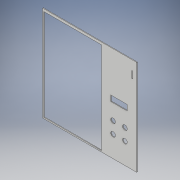
# Autodesk Inventor part: face-avant
Saved by Autodesk Inventor 2019 (Build 230136000, 136)
## iProperties
Created: 2018-12-30
Part Number: face-avant
Material: Générique
Document SubType Name: Modeling
Designer: pouey
Density: 1 g/cm^3
Appearance: Par défaut
Author: pouey
Autodesk Inventor part; units mm, degrees
ref_plane "YZ Plane" through (0, 0, 0) normal (1, 0, 0) x (0, 1, 0)
ref_plane "XZ Plane" through (0, 0, 0) normal (0, 1, 0) x (-1, 0, 0)
ref_plane "XY Plane" through (0, 0, 0) normal (0, 0, 1) x (1, 0, 0)
sketch "Esquisse1" plane through (0, 0, 0) normal (0, 0, 1) x (1, 0, 0)
  line L0 (0, 0) -> (400, 0)
  line L1 (400, 0) -> (400, 405)
  line L2 (400, 405) -> (0, 405)
  line L3 (0, 405) -> (0, 0)
  dimension "d0" = 400
  dimension "d1" = 405
  constraints: 8 end point, 2 parallel, 1 horizontal, 1 perpendicular
  measures "d0" distance of L1.end L2.end
  measures "d1" distance of L0.end L1.end
extrude "Extrusion1" add sketch "Esquisse1" along normal blind 3
sketch "Esquisse2" plane through (0, 0, 3) normal (0, 0, 1) x (1, 0, 0)
  line L0 (5, 395) -> (250, 395)
  line L1 (250, 395) -> (250, 5)
  line L2 (250, 5) -> (5, 5)
  line L3 (5, 5) -> (5, 395)
  line L4 (0, 0) -> (400, 0) projected
  line L5 (0, 405) -> (0, 0) projected
  dimension "d4" = 390
  dimension "d5" = 5
  dimension "d6" = 5
  dimension "d7" = 245
  constraints: 8 end point, 2 parallel, 1 horizontal, 1 perpendicular
  measures "d4" distance of L0.end L1.end
  measures "d5" distance between parallel lines of L4 L2
  measures "d6" distance between parallel lines of L5 L3
  measures "d7" distance between parallel lines of L3 L1
extrude "Extrusion2" cut sketch "Esquisse2" against normal blind 3
sketch "Esquisse3" plane through (0, 0, 3) normal (0, 0, 1) x (1, 0, 0)
  line L0 (290, 230) -> (360, 230)
  line L1 (360, 230) -> (360, 206)
  line L2 (360, 206) -> (290, 206)
  line L3 (290, 206) -> (290, 230)
  line L4 (250, 395) -> (250, 5) projected
  line L5 (400, 405) -> (0, 405) projected
  circle A0 centre (300, 140) radius 10
  circle A1 centre (350, 140) radius 10
  circle A2 centre (300, 90) radius 10
  circle A3 centre (350, 90) radius 10
  line L6 (0, 0) -> (400, 0) projected
  dimension "d10" = 24
  dimension "d11" = 70
  dimension "d13" = 40
  dimension "d14" = 175
  dimension "d17" = 20
  dimension "d18" = 20
  dimension "d19" = 20
  dimension "d20" = 20
  dimension "d21" = 50
  dimension "d22" = 100
  dimension "d23" = 140
  dimension "d24" = 140
  dimension "d25" = 50
  dimension "d26" = 90
  dimension "d27" = 90
  dimension "d28" = 100
  constraints: 8 end point, 4 centre point, 2 parallel, 1 horizontal, 1 perpendicular
  measures "d10" distance of L0.end L1.end
  measures "d11" distance of L0.start L0.end
  measures "d13" distance between parallel lines of L4 L3
  measures "d14" distance between parallel lines of L5 L0
  measures "d17" diameter of A0
  measures "d18" diameter of A1
  measures "d19" diameter of A3
  measures "d20" diameter of A2
  measures "d21" distance from line of L4 A0.centre
  measures "d22" distance from line of L4 A1.centre
  measures "d23" distance from line of L6 A1.centre
  measures "d24" distance from line of L6 A0.centre
  measures "d25" distance from line of L4 A2.centre
  measures "d26" distance from line of L6 A2.centre
  measures "d27" distance from line of L6 A3.centre
  measures "d28" distance from line of L4 A3.centre
extrude "Extrusion3" cut sketch "Esquisse3" against normal blind 3
sketch "Esquisse4" plane through (0, 0, 3) normal (0, 0, 1) x (1, 0, 0)
  line L0 (380, 365) -> (383, 365)
  line L1 (383, 365) -> (383, 335)
  line L2 (383, 335) -> (380, 335)
  line L3 (380, 335) -> (380, 365)
  line L4 (250, 395) -> (250, 5) projected
  line L5 (400, 405) -> (0, 405) projected
  point P0 (0, 0)
  dimension "d29" = 30
  dimension "d30" = 3
  dimension "d31" = 130
  dimension "d32" = 40
  constraints: 8 end point, 2 parallel, 1 horizontal, 1 perpendicular
  measures "d29" distance of L0.end L1.end
  measures "d30" distance of L0.start L0.end
  measures "d31" distance between parallel lines of L4 L3
  measures "d32" distance between parallel lines of L5 L0
extrude "Extrusion4" cut sketch "Esquisse4" against normal blind 3
